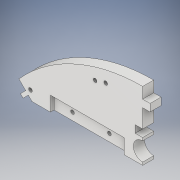
# Autodesk Inventor part: CP005
Saved by Autodesk Inventor 2017 SP1 (Build 210196100, 196)
## iProperties
Created: 2017-05-15
Part Number: CP005
Material: ABS Plastic
Document SubType Name: Modeling
Designer: zallen
Density: 1.06 g/cm^3
Appearance: Smooth - White
Mass: 171.786 g
Surface Area: 320.784 cm^2
Volume: 162.062 cm^3
Author: zallen
Autodesk Inventor part; units mm, degrees
ref_plane "YZ Plane" through (0, 0, 0) normal (1, 0, 0) x (0, 1, 0)
ref_plane "XZ Plane" through (0, 0, 0) normal (0, 1, 0) x (-1, 0, 0)
ref_plane "XY Plane" through (0, 0, 0) normal (0, 0, 1) x (1, 0, 0)
sketch "Sketch1" plane through (0, 0, 0) normal (0, 0, 1) x (1, 0, 0)
  circle A0 centre (0, -132.2876) radius 225 construction
  circle A1 centre (0, -132.2876) radius 200 construction
  line L0 (-225, -132.2876) -> (-150, -132.2876) construction
  line L1 (-150, -132.2876) -> (-150, 35.4175) construction
  line L2 (-175, -132.2876) -> (-175, 9.1338) construction
  arc A2 (0, 92.7124) -> (-167.7086, 17.7086) centre (0, -132.2876) ccw
  line L3 (0, 77.7124) -> (10, 77.7124)
  line L4 (0, 77.7124) -> (10, 77.7124) construction
  line L5 (10, 77.7124) -> (10, 67.7124)
  line L6 (10, 67.7124) -> (0, 67.7124)
  line L7 (0, 67.7124) -> (0, 67.7124)
  line L8 (0, 77.7124) -> (0, 92.7124)
  line L9 (-150, 0) -> (-167.7086, 17.7086)
  line L10 (-150, 0) -> (-124.9563, 0) construction
  line L11 (-150, 0) -> (0, 0)
  line L12 (0, 42.7124) -> (-10, 42.7124)
  line L13 (-10, 42.7124) -> (-10, 32.7124)
  line L14 (-10, 32.7124) -> (0, 32.7124)
  line L15 (0, 67.7124) -> (0, 42.7124)
  line L16 (0, 32.7124) -> (0, 0)
  line L17 (0, -132.2876) -> (0, 252.8934) construction
  dimension "d0" = 450
  dimension "d1" = 25
  dimension "d2" = 75
  dimension "d3" = 25
  dimension "d4" = 10
  dimension "d6" = 10
  dimension "d7" = 15
  dimension "d8" = 135
  dimension "d9" = 10
  dimension "d10" = 10
  dimension "d11" = 25
  dimension "d12" = 90
  dimension "d13" = 90
  dimension "d14" = 90
  constraints: 36 end point, 10 point on circle, 7 point on line, 4 horizontal, 3 centre point, 3 perpendicular, 3 vertical, 2 equal length, 1 coincident, 1 concentric, 1 horizontal alignment, 1 parallel
  measures "d0" diameter of A0
  measures "d1" radial gap between concentric circles of A0 A1
  measures "d2" distance of L0.start L0.end
  measures "d3" distance between parallel lines of L1 L2
  measures "d4" distance of L3.start L3.end
  measures "d6" distance of L3.end L5.end
  measures "d7" distance of L3.start L8.end
  measures "d8" angle of L10 L9
  measures "d9" distance of L12.start L12.end
  measures "d10" distance of L12.end L13.end
  measures "d11" distance of L6.end L12.start
  measures "d12" angle of L5 L6
  measures "d13" angle of L17 L12
  measures "d14" angle of L17 L14
extrude "Extrusion1" add sketch "Sketch1" along normal blind 15
sketch "Sketch3" plane through (0, 0, 15) normal (0, 0, 1) x (1, 0, 0)
  line L0 (-162.0711, -2.0711) -> (-155, 5)
  line L1 (-155, 5) -> (-158.5355, 8.5355)
  line L2 (-158.5355, 8.5355) -> (-165.6066, 1.4645)
  line L3 (-165.6066, 1.4645) -> (-162.0711, -2.0711)
  line L4 (-167.7086, 17.7086) -> (-150, 0) projected
  point P0 (0, 0)
  dimension "d28" = 10
  dimension "d29" = 5
  dimension "d30" = 5
  constraints: 8 end point, 2 parallel, 2 point on line, 1 perpendicular
  measures "d28" distance of L2.end L1.end
  measures "d29" distance of L1.end L0.end
  measures "d30" horizontal distance of L4.end L0.end
extrude "Extrusion2" add sketch "Sketch3" against normal blind 15
sketch "Sketch4" plane through (0, 0, 15) normal (0, 0, 1) x (1, 0, 0)
  circle A0 centre (-64.4318, 67.5838) radius 2.5
  circle A1 centre (-50, 71.6732) radius 2.5
  circle A2 centre (0, -132.2876) radius 225 construction
  arc A3 (0, 92.7124) -> (-167.7086, 17.7086) centre (0, -132.2876) ccw construction
  circle A4 centre (0, -132.2876) radius 210 construction
  circle A5 centre (-152.0028, 12.6094) radius 2.5
  line L0 (-167.7086, 17.7086) -> (-158.5355, 8.5355) projected
  point P0 (0, 0)
  dimension "d33" = 5
  dimension "d34" = 5
  dimension "d35" = 15
  dimension "d36" = 450
  dimension "d37" = 15
  dimension "d38" = 50
  dimension "d45" = 5
  dimension "d49" = 7.5
  constraints: 5 centre point, 3 point on circle, 1 concentric
  measures "d33" diameter of A0
  measures "d34" diameter of A1
  measures "d35" distance of A1.centre A0.centre
  measures "d36" diameter of A2
  measures "d37" radial gap between concentric circles of A2 A4
  measures "d38" horizontal distance of point (0, 0) A1.centre
  measures "d45" diameter of A5
  measures "d49" distance from line of L0 A5.centre
extrude "Extrusion3" cut sketch "Sketch4" against normal through all
thread "Thread1" size "M5x0.8" class "6H" standard "ANSI Metric M Profile" full length
thread "Thread2" size "M5x0.8" class "6H" standard "ANSI Metric M Profile" full length
thread "Thread3" size "M5x0.8" class "6H" standard "ANSI Metric M Profile" full length
sketch "Sketch5" plane through (0, 0, 15) normal (0, 0, 1) x (1, 0, 0)
  line L0 (-150, 0) -> (0, 0) construction
  line L1 (-25, 0) -> (-125, 0) construction
  line L2 (-125, 0) -> (-125, 20) construction
  line L3 (-125, 20) -> (-25, 20) construction
  line L4 (-25, 20) -> (-25, 0) construction
  circle A0 centre (-100, 10) radius 2.5
  circle A1 centre (-50, 10) radius 2.5
  dimension "d52" = 100
  dimension "d53" = 20
  dimension "d54" = 25
  dimension "d55" = 5
  dimension "d56" = 5
  dimension "d57" = 25
  dimension "d58" = 25
  dimension "d59" = 10
  dimension "d60" = 10
  constraints: 8 end point, 2 centre point, 2 parallel, 1 horizontal, 1 perpendicular, 1 point on line
  measures "d52" distance of L2.end L3.end
  measures "d53" distance of L1.end L2.end
  measures "d54" distance of L0.end L1.start
  measures "d55" diameter of A0
  measures "d56" diameter of A1
  measures "d57" distance from line of L2 A0.centre
  measures "d58" distance from line of L4 A1.centre
  measures "d59" distance from line of L0 A0.centre
  measures "d60" distance from line of L0 A1.centre
extrude "Extrusion4" cut sketch "Sketch5" against normal through all
thread "Thread4" size "M5x0.8" class "6H" standard "ANSI Metric M Profile" full length
thread "Thread5" size "M5x0.8" class "6H" standard "ANSI Metric M Profile" full length
sketch "Sketch6" plane through (0, 0, 15) normal (0, 0, 1) x (1, 0, 0)
  line L0 (-125, 0) -> (-25, 0)
  line L1 (-25, 0) -> (-25, 20)
  line L2 (-25, 20) -> (-125, 20)
  line L3 (-125, 20) -> (-125, 0)
  circle A0 centre (-100, 10) radius 2.5 projected
  circle A1 centre (-50, 10) radius 2.5 projected
  line L4 (-162.0711, -2.0711) -> (-155, 5) projected
  line L5 (-155, 5) -> (-150, 0) projected
  line L6 (-150, 0) -> (0, 0) projected
  line L7 (0, 0) -> (0, 32.7124) projected
  line L8 (0, 32.7124) -> (-10, 32.7124) projected
  line L9 (-10, 32.7124) -> (-10, 42.7124) projected
  line L10 (-10, 42.7124) -> (0, 42.7124) projected
  line L11 (0, 42.7124) -> (0, 67.7124) projected
  line L12 (0, 67.7124) -> (10, 67.7124) projected
  line L13 (10, 67.7124) -> (10, 77.7124) projected
  line L14 (10, 77.7124) -> (0, 77.7124) projected
  line L15 (0, 77.7124) -> (0, 92.7124) projected
  arc A2 (0, 92.7124) -> (-167.7086, 17.7086) centre (0, -132.2876) ccw projected
  line L16 (-167.7086, 17.7086) -> (-158.5355, 8.5355) projected
  line L17 (-158.5355, 8.5355) -> (-165.6066, 1.4645) projected
  line L18 (-165.6066, 1.4645) -> (-162.0711, -2.0711) projected
  dimension "d69" = 100
  dimension "d70" = 20
  dimension "d71" = 25
  constraints: 8 end point, 2 parallel, 1 horizontal, 1 perpendicular
  measures "d69" distance of L2.end L1.end
  measures "d70" distance of L1.end L0.end
  measures "d71" distance of L0.start L5.end
extrude "Extrusion5" cut sketch "Sketch6" against normal blind 5 contours L3 L2 L1 L0
sketch "Sketch7" plane through (0, 0, 15) normal (0, 0, 1) x (1, 0, 0)
  line L0 (0, 0) -> (0, 32.7124) projected
  circle A0 centre (0, 16.3562) radius 12.5
  dimension "d74" = 25
  constraints: 1 centre point, 1 midpoint
  measures "d74" diameter of A0
extrude "Extrusion6" cut sketch "Sketch7" against normal through all
body "Solid1"
